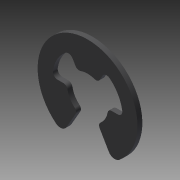
# Autodesk Inventor part: D-5867
Saved by Autodesk Inventor 2014 (Build 180170000, 170)
## iProperties
Created: 2014-01-18
Part Number: D-5867
Material: Steel
Catalog Web Link: www.cadenas.de
Description: Piston Rod Clevis for Original Line Cylinders - Retaining Ring-
Vendor: BIMBA
Document SubType Name: Standard Catalog Part
Designer: Andrew Toennies
Manufacturer: BIMBA
Density: 7.85 g/cm^3
Appearance: Steel
Mass: 1.20987 g
Surface Area: 4.19489 cm^2
Volume: 0.154124 cm^3
Category: PARTsolutions
Company: BIMBA
PSOL_IDENT_0: {$CADENAS_DATA\23d-libs\bimba\bimba\bimba_imperial\bimba_full_line\original_line_cylinders\accessori
PSOL_IDENT_1: es\piston_rod_clevis_rr.prj},210 {VTYP=3D},{NB=D-5867},{LINA=D-5867},{NN=Piston Rod Clevis for Origi
PSOL_IDENT_2: nal Line Cylinders - Retaining Ring},{DATE=06.12.2012 07:53:57},{GEOMDATE=06.12.2012 07:18:40},{VERS
PSOL_IDENT_3: ION=},{LINEID=40},{LINESUBID=-1},{WBVAR=}  {NB=D-5867},{LINA=D-5867},{KT=DUMMY},{PN=D-5867},{D=0.750
PSOL_IDENT_4: 00000},{D1=0.30500000},{D2=0.5275},{L=0.03650000},{COLOR=0.75,0.75,0.75,0.00}
CNS_NN: Piston Rod Clevis for Original Line Cylinders - Retaining Ring
CNS_NB: D-5867
CNS_NBSYN: $PN.
CNS_LINA: D-5867
CNS_PN: D-5867
CNS_D: 0.75000000
CNS_D1: 0.30500000
CNS_D2: 0.527
CNS_L: 0.03650000
CNS_COLOR: 0.75,0.75,0.75,0.00
SUPPLIER: BIMBA
ARTICLENO: D-5867
BOMINFO: D-5867
CREATOR: CADENAS GmbH
Title: D-5867
Author: Cadenas PARTsolutions
Autodesk Inventor part; units mm, degrees
sketch "Sketch_1" plane through (0, 0, 0) normal (0, 0, 1) x (1, 0, 0)
  arc A0 (6.0485, -7.358) -> (-6.0485, -7.358) centre (0, 0) ccw
  arc A1 (-6.0485, -7.358) -> (-4.0374, -6.9929) centre (-5.1977, -6.323) ccw
  line L0 (-4.0374, -6.9929) -> (-2.2916, -3.9692)
  arc A2 (-2.2916, -3.9692) -> (-2.4688, -2.9848) centre (-2.9625, -3.5818) ccw
  arc A3 (-3.8193, -0.6456) -> (-2.4688, -2.9848) centre (0, 0) ccw
  arc A4 (-3.8193, -0.6456) -> (-4.5832, 0) centre (-4.5832, -0.7747) ccw
  line L1 (-4.5832, 0) -> (-5.7369, 0)
  arc A5 (-6.6195, 1.0307) -> (-5.7369, 0) centre (-5.7369, 0.8932) ccw
  arc A6 (-4.2023, 5.2173) -> (-6.6195, 1.0307) centre (0, 0) ccw
  arc A7 (-2.8684, 4.9683) -> (-4.2023, 5.2173) centre (-3.642, 4.5217) ccw
  line L2 (-2.8684, 4.9683) -> (-2.2916, 3.9692)
  arc A8 (-2.2916, 3.9692) -> (-1.3506, 3.6304) centre (-1.6207, 4.3565) ccw
  arc A9 (1.3506, 3.6304) -> (-1.3506, 3.6304) centre (0, 0) ccw
  arc A10 (1.3506, 3.6304) -> (2.2916, 3.9692) centre (1.6207, 4.3565) ccw
  line L3 (2.2916, 3.9692) -> (2.8684, 4.9683)
  arc A11 (4.2023, 5.2173) -> (2.8684, 4.9683) centre (3.642, 4.5217) ccw
  arc A12 (6.6195, 1.0307) -> (4.2023, 5.2173) centre (0, 0) ccw
  arc A13 (5.7369, 0) -> (6.6195, 1.0307) centre (5.7369, 0.8932) ccw
  line L4 (5.7369, 0) -> (4.5832, 0)
  arc A14 (4.5832, 0) -> (3.8193, -0.6456) centre (4.5832, -0.7747) ccw
  arc A15 (2.4688, -2.9848) -> (3.8193, -0.6456) centre (0, 0) ccw
  arc A16 (2.4688, -2.9848) -> (2.2916, -3.9692) centre (2.9625, -3.5818) ccw
  line L5 (2.2916, -3.9692) -> (4.0374, -6.9929)
  arc A17 (4.0374, -6.9929) -> (6.0485, -7.358) centre (5.1977, -6.323) ccw
  constraints: 36 point on circle, 18 centre point, 12 end point
extrude "Extrusion1" add sketch "Sketch_1" along normal mid plane 0.9271
ref_plane "RR_XY" through (0, 0, 0) normal (0, 0, 1) x (1, 0, 0)
ref_plane "RR_YZ" through (0, 0, 0) normal (1, 0, 0) x (0, 1, 0)
ref_plane "RR_ZX" through (0, 0, 0) normal (0, 1, 0) x (0, 0, 1)
body "Solid1"
